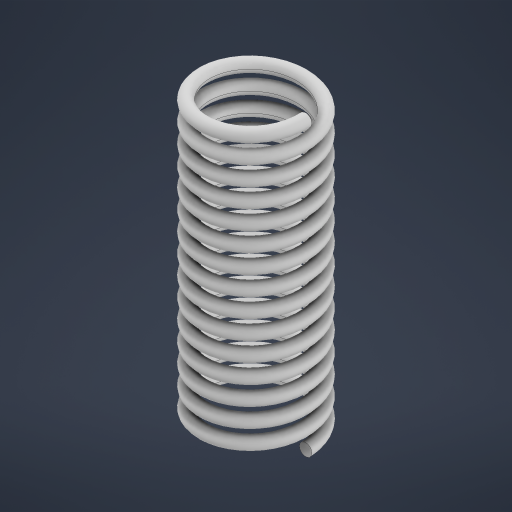
# Autodesk Inventor part: sf_Pivot_Shaft_Spring_1
Saved by Autodesk Inventor 2024 (Build 280153000, 153)
## iProperties
Created: 2024-03-22
Part Number: sf_Pivot_Shaft_Spring_1
Material: Generisch
Document SubType Name: Modeling
Designer: Simon
Density: 1 g/cm^3
Appearance: Vorgabe
Author: Simon
Autodesk Inventor part; units mm, degrees
ref_plane "YZ Plane" through (0, 0, 0) normal (1, 0, 0) x (0, 1, 0)
ref_plane "XZ Plane" through (0, 0, 0) normal (0, 1, 0) x (-1, 0, 0)
ref_plane "XY Plane" through (0, 0, 0) normal (0, 0, 1) x (1, 0, 0)
sketch "Skizze1" plane through (0, 0, 0) normal (0, 1, 0) x (-1, 0, 0)
  circle A0 centre (-4, 0) radius 0.5
  line L0 (0, 0) -> (0, 0.7995) construction
  point P0 (-3.5, 0)
  dimension "d0" = 1
  dimension "d1" = 4
  dimension "d2" = 3.5
  constraints: 2 end point, 1 horizontal alignment, 1 vertical, 2 other
  measures "d1" distance of L0.start point (-4, 0)
  measures "d2" distance of L0.start point (-3.5, 0)
coil "Spirale1" sketch "Skizze1" operation add axis through (0, 0, 0) along (0, 0, 1) pitch 1.5333 turns 15 hand right
